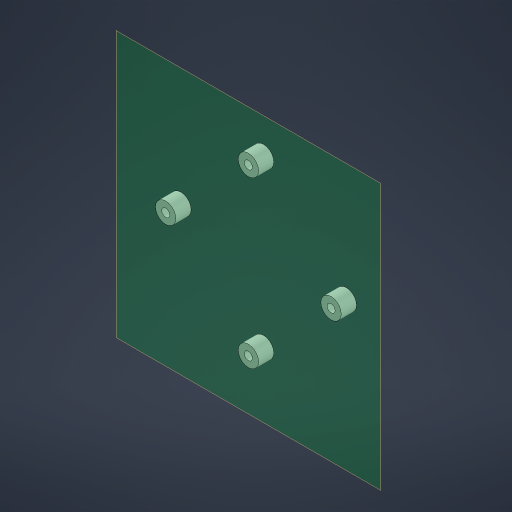
# Autodesk Inventor part: OmniFrame_C
Saved by Autodesk Inventor 2024.2 (Build 282272000, 272)
## iProperties
Created: 2024-02-19
Part Number: OmniFrame_C
Material: 一般
Document SubType Name: Modeling
Designer: Hanaoka
Density: 1 g/cm^3
Appearance: 既定
Author: Hanaoka
Autodesk Inventor part; units mm, degrees
ref_plane "YZ Plane" through (0, 0, 0) normal (1, 0, 0) x (0, 1, 0)
ref_plane "XZ Plane" through (0, 0, 0) normal (0, 1, 0) x (-1, 0, 0)
ref_plane "XY Plane" through (0, 0, 0) normal (0, 0, 1) x (1, 0, 0)
ref_plane "作業平面1" through (27.8985, 22.9434, -0.1984) normal (0, 0, -1) x (0, -1, 0)
sketch "スケッチ1" plane through (27.8985, 22.9434, -0.1984) normal (0, 0, -1) x (0, -1, 0)
  circle A0 centre (-16.25, 0) radius 0.8 projected
  circle A1 centre (0, -16.25) radius 0.8 projected
  circle A2 centre (16.25, 0) radius 0.8 projected
  circle A3 centre (0, 16.25) radius 0.8 projected
  circle A4 centre (-16.25, 0) radius 2
  circle A5 centre (0, 16.25) radius 2
  circle A6 centre (0, -16.25) radius 2
  circle A7 centre (16.25, 0) radius 2
  point P0 (22.9434, 27.8985)
  dimension "d0" = 4
  constraints: 4 centre point, 4 coincident, 3 equal radius
  measures "d0" diameter of A4
extrude "押し出し1" add sketch "スケッチ1" along normal blind 3
